Autodesk Inventor part; units mm, degrees
(part 2 of 2)
sketch "Sketch8" plane through (115, 30, -7.5) normal (0, 0, -1) x (-1, 0, 0)
  circle A0 centre (-27.5, -0.5) radius 2.15
  circle A1 centre (-27.5, -59.5) radius 2.15
  arc A2 (-24.035898, 1.5) -> (-26.5, -4.372983) centre (-27.5, -0.5) ccw
  line L0 (-26.5, -4.372983) -> (-26.5, -55.627017)
  arc A3 (-26.5, -55.627017) -> (-24.035898, -61.5) centre (-27.5, -59.5) ccw
  line L1 (-24.035898, -61.5) -> (41.5, -61.5)
  line L2 (41.5, -61.5) -> (41.5, 1.5)
  line L3 (41.5, 1.5) -> (-24.035898, 1.5)
  line L4 (16.06066, -5) -> (13.03033, -1.96967)
  line L5 (13.03033, -1.96967) -> (15, 0)
  line L6 (15, 0) -> (35, 0)
  line L7 (35, 0) -> (36.96967, -1.96967)
  line L8 (36.96967, -1.96967) -> (33.93934, -5)
  line L9 (33.93934, -5) -> (16.06066, -5)
  line L10 (11.96967, -3.03033) -> (15, -6.06066)
  line L11 (15, -6.06066) -> (15, -26.43934)
  line L12 (15, -26.43934) -> (12.5, -28.93934)
  line L13 (12.5, -28.93934) -> (10, -26.43934)
  line L14 (10, -26.43934) -> (10, -5)
  line L15 (10, -5) -> (11.96967, -3.03033)
  line L16 (16.06066, -27.5) -> (33.93934, -27.5)
  line L17 (33.93934, -27.5) -> (36.43934, -30)
  line L18 (36.43934, -30) -> (33.93934, -32.5)
  line L19 (33.93934, -32.5) -> (16.06066, -32.5)
  line L20 (16.06066, -32.5) -> (13.56066, -30)
  line L21 (13.56066, -30) -> (16.06066, -27.5)
  line L22 (38.03033, -56.96967) -> (35, -53.93934)
  line L23 (35, -53.93934) -> (35, -33.56066)
  line L24 (35, -33.56066) -> (37.5, -31.06066)
  line L25 (37.5, -31.06066) -> (40, -33.56066)
  line L26 (40, -33.56066) -> (40, -55)
  line L27 (40, -55) -> (38.03033, -56.96967)
  line L28 (13.03033, -58.03033) -> (16.06066, -55)
  line L29 (16.06066, -55) -> (33.93934, -55)
  line L30 (33.93934, -55) -> (36.96967, -58.03033)
  line L31 (36.96967, -58.03033) -> (35, -60)
  line L32 (35, -60) -> (15, -60)
  line L33 (15, -60) -> (13.03033, -58.03033)
  line L34 (15, -53.93934) -> (11.96967, -56.96967)
  line L35 (11.96967, -56.96967) -> (10, -55)
  line L36 (10, -55) -> (10, -33.56066)
  line L37 (10, -33.56066) -> (12.5, -31.06066)
  line L38 (12.5, -31.06066) -> (15, -33.56066)
  line L39 (15, -33.56066) -> (15, -53.93934)
  line L40 (3.03033, -56.96967) -> (0, -53.93934)
  line L41 (0, -53.93934) -> (0, -33.56066)
  line L42 (0, -33.56066) -> (2.5, -31.06066)
  line L43 (2.5, -31.06066) -> (5, -33.56066)
  line L44 (5, -33.56066) -> (5, -55)
  line L45 (5, -55) -> (3.03033, -56.96967)
  line L46 (-18.93934, -27.5) -> (-1.06066, -27.5)
  line L47 (-1.06066, -27.5) -> (1.43934, -30)
  line L48 (1.43934, -30) -> (-1.06066, -32.5)
  line L49 (-1.06066, -32.5) -> (-18.93934, -32.5)
  line L50 (-18.93934, -32.5) -> (-21.43934, -30)
  line L51 (-21.43934, -30) -> (-18.93934, -27.5)
  line L52 (0, -6.06066) -> (3.03033, -3.03033)
  line L53 (3.03033, -3.03033) -> (5, -5)
  line L54 (5, -5) -> (5, -26.43934)
  line L55 (5, -26.43934) -> (2.5, -28.93934)
  line L56 (2.5, -28.93934) -> (0, -26.43934)
  line L57 (0, -26.43934) -> (0, -6.06066)
  line L58 (-18.93934, -5) -> (-21.96967, -1.96967)
  line L59 (-21.96967, -1.96967) -> (-20, 0)
  line L60 (-20, 0) -> (0, 0)
  line L61 (0, 0) -> (1.96967, -1.96967)
  line L62 (1.96967, -1.96967) -> (-1.06066, -5)
  line L63 (-1.06066, -5) -> (-18.93934, -5)
  line L64 (-20, -53.93934) -> (-23.03033, -56.96967)
  line L65 (-23.03033, -56.96967) -> (-25, -55)
  line L66 (-25, -55) -> (-25, -33.56066)
  line L67 (-25, -33.56066) -> (-22.5, -31.06066)
  line L68 (-22.5, -31.06066) -> (-20, -33.56066)
  line L69 (-20, -33.56066) -> (-20, -53.93934)
  line L70 (-21.96967, -58.03033) -> (-18.93934, -55)
  line L71 (-18.93934, -55) -> (-1.06066, -55)
  line L72 (-1.06066, -55) -> (1.96967, -58.03033)
  line L73 (1.96967, -58.03033) -> (0, -60)
  line L74 (0, -60) -> (-20, -60)
  line L75 (-20, -60) -> (-21.96967, -58.03033)
  line L76 (38.03033, -3.03033) -> (40, -5)
  line L77 (40, -5) -> (40, -26.43934)
  line L78 (40, -26.43934) -> (37.5, -28.93934)
  line L79 (37.5, -28.93934) -> (35, -26.43934)
  line L80 (35, -26.43934) -> (35, -6.06066)
  line L81 (35, -6.06066) -> (38.03033, -3.03033)
  line L82 (-22.5, -28.93934) -> (-25, -26.43934)
  line L83 (-25, -26.43934) -> (-25, -5)
  line L84 (-25, -5) -> (-23.03033, -3.03033)
  line L85 (-23.03033, -3.03033) -> (-20, -6.06066)
  line L86 (-20, -6.06066) -> (-20, -26.43934)
  line L87 (-20, -26.43934) -> (-22.5, -28.93934)
  line L88 (33.5, -6.5) -> (33.5, -26)
  line L89 (33.5, -26) -> (16.5, -26)
  line L90 (16.5, -26) -> (16.5, -6.5)
  line L91 (16.5, -6.5) -> (33.5, -6.5)
  line L92 (-1.5, -6.5) -> (-1.5, -26)
  line L93 (-1.5, -26) -> (-18.5, -26)
  line L94 (-18.5, -26) -> (-18.5, -6.5)
  line L95 (-18.5, -6.5) -> (-1.5, -6.5)
  line L96 (33.5, -53.5) -> (16.5, -53.5)
  line L97 (16.5, -53.5) -> (16.5, -34)
  line L98 (16.5, -34) -> (33.5, -34)
  line L99 (33.5, -34) -> (33.5, -53.5)
  line L100 (-1.5, -53.5) -> (-18.5, -53.5)
  line L101 (-18.5, -53.5) -> (-18.5, -34)
  line L102 (-18.5, -34) -> (-1.5, -34)
  line L103 (-1.5, -34) -> (-1.5, -53.5)
  circle A4 centre (52.5, -0.5) radius 4
  circle A5 centre (52.5, -0.5) radius 2.15
  circle A6 centre (52.5, -15.71967) radius 4
  circle A7 centre (52.5, -15.71967) radius 2.5
  circle A8 centre (52.5, -44.28033) radius 2.5
  circle A9 centre (52.5, -44.28033) radius 4
  circle A10 centre (52.5, -59.5) radius 4
  circle A11 centre (52.5, -59.5) radius 2.15
  line L104 (-31.5, 3.5) -> (56.5, 3.5)
  line L105 (56.5, 3.5) -> (56.5, -63.5)
  line L106 (56.5, -63.5) -> (-31.5, -63.5)
  line L107 (-31.5, -63.5) -> (-31.5, 3.5)
  circle A12 centre (52.5, -59.5) radius 4
  arc A13 (-24.035898, 1.5) -> (-26.5, -4.372983) centre (-27.5, -0.5) ccw
  line L108 (-15.5, -5) -> (-4.5, -5)
  line L109 (-4.5, -5) -> (-4.5, 0)
  line L110 (-4.5, 0) -> (-15.5, 0)
  line L111 (-15.5, 0) -> (-15.5, -5)
  circle A14 centre (-15.5, -2.5) radius 2
  circle A15 centre (-4.5, -2.5) radius 2
  line L112 (30.5, -5) -> (30.5, 0)
  line L113 (19.5, -5) -> (30.5, -5)
  line L114 (30.5, 0) -> (19.5, 0)
  line L115 (19.5, 0) -> (19.5, -5)
  circle A16 centre (19.5, -2.5) radius 2
  circle A17 centre (30.5, -2.5) radius 2
  line L116 (-4.5, -32.5) -> (-4.5, -27.5)
  line L117 (-15.5, -32.5) -> (-4.5, -32.5)
  line L118 (-4.5, -27.5) -> (-15.5, -27.5)
  line L119 (-15.5, -27.5) -> (-15.5, -32.5)
  circle A18 centre (-15.5, -30) radius 2
  circle A19 centre (-4.5, -30) radius 2
  line L120 (30.5, -32.5) -> (30.5, -27.5)
  line L121 (19.5, -32.5) -> (30.5, -32.5)
  line L122 (30.5, -27.5) -> (19.5, -27.5)
  line L123 (19.5, -27.5) -> (19.5, -32.5)
  circle A20 centre (19.5, -30) radius 2
  circle A21 centre (30.5, -30) radius 2
  line L124 (-4.5, -60) -> (-4.5, -55)
  line L125 (-15.5, -60) -> (-4.5, -60)
  line L126 (-4.5, -55) -> (-15.5, -55)
  line L127 (-15.5, -55) -> (-15.5, -60)
  circle A22 centre (-15.5, -57.5) radius 2
  circle A23 centre (-4.5, -57.5) radius 2
  line L128 (30.5, -60) -> (30.5, -55)
  line L129 (19.5, -60) -> (30.5, -60)
  line L130 (30.5, -55) -> (19.5, -55)
  line L131 (19.5, -55) -> (19.5, -60)
  circle A24 centre (19.5, -57.5) radius 2
  circle A25 centre (30.5, -57.5) radius 2
  line L132 (-20, -26.43934) -> (-20, -6.06066)
  line L133 (-25, -9.21967) -> (-20, -9.21967)
  line L134 (-20, -9.21967) -> (-20, -22.21967)
  line L135 (-20, -22.21967) -> (-25, -22.21967)
  line L136 (-25, -22.21967) -> (-25, -9.21967)
  circle A26 centre (-22.5, -9.21967) radius 2
  circle A27 centre (-22.5, -22.21967) radius 2
  circle A28 centre (-22.5, -37.78067) radius 2
  circle A29 centre (-22.5, -50.78067) radius 2
  circle A30 centre (2.522, -9.21967) radius 2
  circle A31 centre (2.522, -22.21967) radius 2
  circle A32 centre (2.522, -37.78067) radius 2
  circle A33 centre (2.522, -50.78067) radius 2
  circle A34 centre (37.522, -22.21967) radius 2
  circle A35 centre (12.5, -9.21967) radius 2
  circle A36 centre (37.522, -9.21967) radius 2
  circle A37 centre (12.5, -22.21967) radius 2
  circle A38 centre (12.5, -37.78067) radius 2
  circle A39 centre (12.5, -50.78067) radius 2
  circle A40 centre (37.522, -37.78067) radius 2
  circle A41 centre (37.522, -50.78067) radius 2
  line L137 (-22.5, -9.21967) -> (-22.5, -22.21967)
  line L138 (-15.5, -2.5) -> (-4.5, -2.5)
  line L139 (-22.5, -37.78067) -> (-22.5, -50.78067)
  line L140 (-15.5, -30) -> (-4.5, -30)
  line L141 (2.522, -9.21967) -> (2.522, -22.21967)
  line L142 (2.522, -37.78067) -> (2.522, -50.78067)
  line L143 (-15.5, -57.5) -> (-4.5, -57.5)
  circle A42 centre (-22.5, -15.71967) radius 1.5
  circle A43 centre (-10, -2.5) radius 1.5
  circle A44 centre (2.522, -15.71967) radius 1.5
  circle A45 centre (-22.5, -44.28067) radius 1.5
  circle A46 centre (2.522, -44.28067) radius 1.5
  circle A47 centre (-10, -30) radius 1.5
  circle A48 centre (-10, -57.5) radius 1.5
  circle A49 centre (12.5, -15.71967) radius 1.5
  circle A50 centre (25, -2.5) radius 1.5
  circle A51 centre (37.522, -15.71967) radius 1.5
  circle A52 centre (25, -30) radius 1.5
  circle A53 centre (12.5, -44.28067) radius 1.5
  circle A54 centre (25, -57.5) radius 1.5
  circle A55 centre (37.522, -44.28067) radius 1.5
  point P0 (115, -30)
  point P1 (-10, 0)
  point P2 (25, 0)
  point P3 (-10, -27.5)
  point P4 (25, -27.5)
  point P5 (-10, -55)
  point P6 (25, -55)
  point P7 (-25, -15.71967)
  dimension "d141" = 22.87868
  dimension "d142" = 25.90901
  dimension "d143" = 11
  dimension "d144" = 4
  dimension "d145" = 4
  dimension "d148" = 35
  dimension "d151" = 27.5
  dimension "d161" = 13
  dimension "d162" = 4
  dimension "d163" = 4
  dimension "d166" = 28.561
  dimension "d169" = 25.022
  dimension "d174" = 35
  dimension "d186" = 3
  dimension "d187" = 3
  dimension "d188" = 3
  dimension "d189" = 3
  dimension "d190" = 3
  dimension "d191" = 3
  dimension "d192" = 3
  dimension "d195" = 35
  dimension "d200" = 88
  dimension "d201" = 67
  dimension "d221" = 5
  dimension "d222" = 20
  dimension "d223" = 22.5
  constraints: 78 end point, 42 centre point, 15 midpoint, 8 coincident, 8 horizontal, 8 parallel, 5 vertical, 4 perpendicular, 4 point on line, 4 tangent, 112 other
  measures "d141" distance of L50.end L47.end
  measures "d142" vertical distance of L84.end L82.start
  measures "d143" distance from line of L109 point (-15.5, -2.5)
  measures "d144" diameter of A14
  measures "d145" diameter of A15
  measures "d148" distance of L109.end L112.end
  measures "d151" distance of L109.end L116.end
  measures "d161" distance of point (-22.5, -9.22) point (-22.5, -22.22)
  measures "d162" diameter of A26
  measures "d163" diameter of A27
  measures "d166" distance of L137.start L139.start
  measures "d169" distance of L137.start L141.start
  measures "d174" distance of L141.end A34.centre
  measures "d186" diameter of A42
  measures "d187" diameter of A43
  measures "d188" diameter of A44
  measures "d189" diameter of A45
  measures "d190" diameter of A46
  measures "d191" diameter of A47
  measures "d192" diameter of A48
  measures "d195" distance of A42.centre A49.centre
  measures "d200" distance of L104.start L104.end
  measures "d201" distance of L104.end L105.end
  measures "d221" distance between parallel lines of L77 L80
  measures "d222" distance between parallel lines of L11 L80
  measures "d223" distance between parallel lines of L16 L9
fillet "Fillet1" radius 4 6 edges at (73.5, 31.5, -4) (-16.5, 31.5, -4) (-16.5, -31.5, -4) (73.5, -31.5, -4) (163.5, 31.5, -4) (163.5, -31.5, -4)
equation "\"d121\" = bobyshka_d"
equation "\"d123\" = bobyshka_d"
equation "\"d125\" = bobyshka_d"
body "Solid1"
